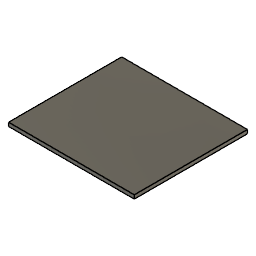
PCB (Autodesk Fusion 360 design; units mm, degrees)
part number: 2026-03-31-20-07-59-001
Autodesk Fusion 360 part; units mm, degrees
sketch "Boceto1" plane through (0, 0, 0) normal (0, 0, 1) x (1, 0, 0)
  line L0 (50, -45) -> (-50, -45)
  line L1 (-50, -45) -> (-50, 45)
  line L2 (-50, 45) -> (50, 45)
  line L3 (50, 45) -> (50, -45)
  line L4 (50, -45) -> (-50, 45) construction
  line L5 (-50, -45) -> (50, 45) construction
  dimension "d1" = 100
  dimension "d2" = 90
  constraint horizontal L0
  constraint perpendicular L0 L1
  constraint parallel L0 L2
  constraint parallel L1 L3
  constraint coincident L4 origin
  constraint coincident L5 origin
  measures "d1" distance of L1.end L2.end
  measures "d2" distance of L0.end L1.end
extrude "Extruir1" add sketch "Boceto1" along normal blind 3
